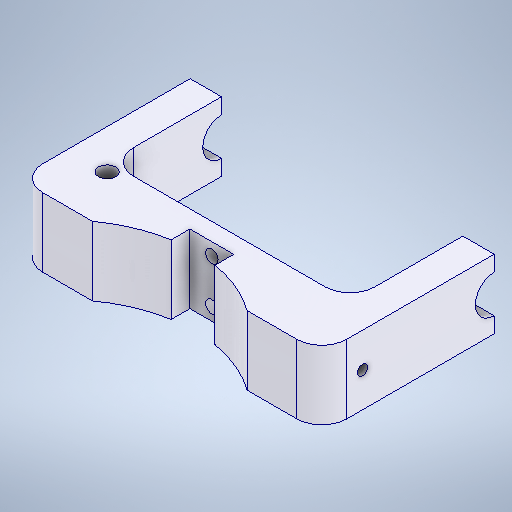
# Autodesk Inventor part: 145 part 2
Saved by Autodesk Inventor 2025.1 (Build 291241000, 241)
## iProperties
Created: 2024-08-01
Part Number: 145 part 2
Material: Aluminum 6061-AHC
Document SubType Name: Modeling
Designer: ffogue
Density: 2.7 g/cm^3
Appearance: Cool White
Author: ffogue
Autodesk Inventor part; units mm, degrees
note: some values were not read from the file. Chosen so that the rebuilt part matches the saved one: direction of "Hole1".
ref_plane "YZ Plane" through (0, 0, 0) normal (1, 0, 0) x (0, 1, 0)
ref_plane "XZ Plane" through (0, 0, 0) normal (0, 1, 0) x (-1, 0, 0)
ref_plane "XY Plane" through (0, 0, 0) normal (0, 0, 1) x (1, 0, 0)
sketch "Sketch1" plane through (0, 0, 0) normal (0, 0, 1) x (1, 0, 0)
  line L0 (-48.5, 0) -> (-48.5, 55)
  line L1 (-48.5, 55) -> (-38.5, 55)
  line L2 (-38.5, 55) -> (-38.5, 27)
  line L3 (-30.5, 19) -> (30.5, 19)
  line L4 (38.5, 27) -> (38.5, 55)
  line L5 (38.5, 55) -> (48.5, 55)
  line L6 (48.5, 55) -> (48.5, 0)
  line L7 (48.5, 0) -> (-48.5, 0)
  arc A0 (-38.5, 27) -> (-30.5, 19) centre (-30.5, 27) ccw
  arc A1 (30.5, 19) -> (38.5, 27) centre (30.5, 27) ccw
  line L8 (0, 0) -> (0, 59.4805) construction
  point P0 (0, 0)
  point P1 (0, 19)
  dimension "d0" = 10
  dimension "d1" = 19
  dimension "d2" = 36
  dimension "d3" = 8
  dimension "d4" = 97
  constraints: 18 end point, 6 perpendicular, 4 point on circle, 4 tangent, 2 centre point, 2 midpoint, 2 point on line, 2 vertical, 1 coincident, 1 equal radius, 1 horizontal alignment, 1 symmetric about line, 1 vertical alignment
  measures "d0" distance between parallel lines of L2 L0
  measures "d1" distance between parallel lines of L7 L3
  measures "d2" distance between parallel lines of L3 L1
  measures "d3" radius of A0
  measures "d4" distance between parallel lines of L6 L0
extrude "Extrusion1" add sketch "Sketch1" against normal blind 22
sketch "Sketch2" plane through (0, 0, 0) normal (0, 0, 1) x (1, 0, 0)
  arc A0 (24.6577, 0) -> (-24.6577, 0) centre (0, -34) ccw
  line L0 (-48.5, 0) -> (48.5, 0) projected
  line L1 (-24.6577, 0) -> (24.6577, 0)
  point P0 (0, 0)
  point P1 (0, 0)
  point P2 (0, 0)
  point P3 (-24.6577, 0)
  point P4 (24.6577, 0)
  dimension "d7" = 84
  dimension "d8" = 8
  constraints: 3 midpoint, 2 end point, 2 point on circle, 1 centre point, 1 coincident, 1 horizontal
  measures "d7" diameter of A0
  measures "d8" distance edge to line of A0 L1
extrude "Extrusion2" cut sketch "Sketch2" against normal up to surface (22 mm away)
sketch "Sketch3" plane through (0, 0, 0) normal (0, 0, 1) x (1, 0, 0)
  arc A0 (24.6577, 0) -> (-24.6577, 0) centre (0, -34) ccw projected
  line L0 (-7, 7.4126) -> (-7, 13.4126)
  line L1 (-7, 13.4126) -> (7, 13.4126)
  line L2 (7, 13.4126) -> (7, 7.4126)
  line L3 (0, 0) -> (0, 19) construction
  line L4 (30.5, 19) -> (-30.5, 19) projected
  dimension "d11" = 14
  dimension "d12" = 6
  constraints: 8 end point, 2 perpendicular, 2 point on circle, 1 midpoint, 1 vertical, 1 other
  measures "d11" distance between parallel lines of L2 L0
  measures "d12" distance of L0.start L0.end
extrude "Extrusion3" cut sketch "Sketch3" against normal up to surface (22 mm away)
sketch "Sketch4" plane through (0, 0, 0) normal (0, 0, 1) x (1, 0, 0)
  line L0 (-48.5, 55) -> (-48.5, 0) projected
  line L1 (-48.5, 0) -> (-24.6577, 0) projected
  point P0 (0, 0)
  point P1 (-36, 16)
  dimension "d22" = 12.5
  dimension "d23" = 16
  measures "d22" distance from line of L0 point (-36, 16)
  measures "d23" distance from line of L1 point (-36, 16)
hole "Hole1" at (-36, 16, 0) direction (0, 0, -1) diameter 5.5 depth 22
sketch "Sketch5" plane through (-48.5, 0, 0) normal (-1, 0, 0) x (0, 0, 1)
  line L0 (0, 55) -> (-22, 55) projected
  arc A0 (-17, 55) -> (-5, 55) centre (-11, 55) ccw
  line L1 (-17, 55) -> (-5, 55)
  point P0 (0, 0)
  point P1 (-5, 55)
  dimension "d24" = 12
  constraints: 3 midpoint, 2 end point, 2 point on circle, 1 centre point, 1 coincident, 1 horizontal
  measures "d24" diameter of A0
extrude "Extrusion4" cut sketch "Sketch5" against normal up to surface (10 mm away)
mirror "Mirror1" about plane through (0, 0, 0) normal (1, 0, 0) of "Extrusion4"
sketch "Sketch6" plane through (-48.5, 55, 0) normal (0, 1, 0) x (1, 0, 0)
  line L0 (0, 5) -> (0, 17) projected
  line L1 (0, 22) -> (10, 22) projected
  point P0 (48.5, 0)
  point P1 (5, 19)
  point P2 (5, 3)
  point P3 (0, 11)
  point P4 (5, 22)
  dimension "d27" = 8
  dimension "d28" = 8
  constraints: 2 midpoint, 2 vertical alignment
  measures "d27" vertical distance of point (0, 11) point (5, 3)
  measures "d28" vertical distance of point (0, 11) point (5, 19)
hole "Hole2" at (-43.5, 55, -19) at (-43.5, 55, -3) direction (0, -1, 0) diameter 3 depth 5
mirror "Mirror2" about plane through (0, 0, 0) normal (1, 0, 0) of "Hole2"
fillet "Fillet1" radius 8 2 edges at (48.5, 0, -11) (-48.5, 0, -11)
sketch "Sketch7" plane through (48.5, 55, -11) normal (1, 0, 0) x (0, 0, -1)
  line L0 (-11, -55) -> (11, -55) projected
  point P0 (0, -42)
  point P1 (0, -55)
  dimension "d44" = 13
  constraints: 1 midpoint, 1 vertical alignment
  measures "d44" distance from line of L0 point (0, -42)
hole "Hole3" at (48.5, 13, -11) direction (-1, 0, 0) diameter 3.242 depth 19 thread size "M4x0.7" class "6H" standard "ISO Metric profile"
sketch "Sketch8" plane through (-30.5, 19, 0) normal (0, 1, 0) x (1, 0, 0)
  line L0 (-8, 17) -> (-8, 5) projected
  circle A0 centre (-13, 3) radius 1.5 projected
  circle A1 centre (-13, 19) radius 1.5 projected
  point P0 (30.5, 0)
  point P1 (30.5, 18)
  point P2 (30.5, 4)
  point P3 (-8, 11)
  dimension "d52" = 7
  dimension "d53" = 7
  dimension "d54" = 43.5
  dimension "d55" = 43.5
  constraints: 1 midpoint, 1 vertical alignment
  measures "d52" vertical distance of point (-8, 11) point (30.5, 18)
  measures "d53" vertical distance of point (-8, 11) point (30.5, 4)
  measures "d54" horizontal distance of point (30.5, 4) A0.centre
  measures "d55" horizontal distance of A1.centre point (30.5, 18)
hole "Hole4" at (0, 19, -18) at (0, 19, -4) direction (0, -1, 0) diameter 4 end through all
sketch "Skizze9" plane through (0, 0, 0) normal (0, 0, 1) x (1, 0, 0)
  circle A0 centre (-36, 16) radius 2.75 projected
  arc A1 (-48.5, 8) -> (-40.5, 0) centre (-40.5, 8) ccw projected
  line L0 (-40.5, 0) -> (-24.6577, 0) projected
  arc A2 (-7, 7.4126) -> (-24.6577, 0) centre (0, -34) ccw projected
  line L1 (-7, 7.4126) -> (-7, 13.4126) projected
  line L2 (-7, 13.4126) -> (7, 13.4126) projected
  line L3 (7, 13.4126) -> (7, 7.4126) projected
  arc A3 (24.6577, 0) -> (7, 7.4126) centre (0, -34) ccw projected
  line L4 (24.6577, 0) -> (40.5, 0) projected
  arc A4 (40.5, 0) -> (48.5, 8) centre (40.5, 8) ccw projected
  line L5 (48.5, 8) -> (48.5, 55) projected
  line L6 (48.5, 55) -> (38.5, 55) projected
  line L7 (38.5, 55) -> (38.5, 27) projected
  arc A5 (30.5, 19) -> (38.5, 27) centre (30.5, 27) ccw projected
  line L8 (30.5, 19) -> (-30.5, 19) projected
  arc A6 (-38.5, 27) -> (-30.5, 19) centre (-30.5, 27) ccw projected
  line L9 (-38.5, 27) -> (-38.5, 55) projected
  line L10 (-38.5, 55) -> (-48.5, 55) projected
  line L11 (-48.5, 55) -> (-48.5, 8) projected
  arc A7 (24.6577, 0) -> (-24.6577, 0) centre (0, -34) ccw
  point P0 (0, 0)
  constraints: 2 point on circle, 1 centre point, 1 concentric
equation "\"d28\" = d27"
equation "\"d53\" = d52"
body "Solid1"
